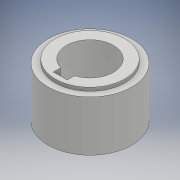
# Autodesk Inventor part: Outer Wheel Spacer
Saved by Autodesk Inventor 2018 (Build 220112000, 112)
## iProperties
Created: 2018-01-21
Part Number: Outer Wheel Spacer
Material: Generic
Document SubType Name: Modeling
Designer: Apple
Density: 1 g/cm^3
Appearance: Default
Author: Apple
Autodesk Inventor part; units mm, degrees
ref_plane "YZ Plane" through (0, 0, 0) normal (1, 0, 0) x (0, 1, 0)
ref_plane "XZ Plane" through (0, 0, 0) normal (0, 1, 0) x (-1, 0, 0)
ref_plane "XY Plane" through (0, 0, 0) normal (0, 0, 1) x (1, 0, 0)
sketch "Sketch1" plane through (0, 0, 0) normal (0, 0, 1) x (1, 0, 0)
  circle A0 centre (0, 0) radius 6.75
  circle A1 centre (0, 0) radius 12
  dimension "d0" = 13.5
  dimension "d1" = 24
  constraints: 2 centre point, 2 coincident
  measures "d0" diameter of A0
  measures "d1" diameter of A1
extrude "Extrusion1" add sketch "Sketch1" along normal blind 14.5
sketch "Sketch3" plane through (0, 0, 14.5) normal (0, 0, 1) x (1, 0, 0)
  circle A0 centre (0, 0) radius 10
  circle A1 centre (0, 0) radius 6.75 projected
  dimension "d7" = 20
  constraints: 1 centre point, 1 coincident
  measures "d7" diameter of A0
extrude "Extrusion3" add sketch "Sketch3" along normal blind 1
sketch "Sketch5" plane through (0, 0, 15.5) normal (0, 0, 1) x (1, 0, 0)
  line L0 (2, -8.55) -> (-2, -8.55)
  line L1 (-2, -8.55) -> (-2, -4.55)
  line L2 (-2, -4.55) -> (2, -4.55)
  line L3 (2, -4.55) -> (2, -8.55)
  line L4 (3.7816, -6.55) -> (-3.7816, -6.55) projected
  point P0 (0, 0)
  point P1 (0, -8.55)
  point P2 (-2, -6.55)
  point P3 (0, -6.55)
  dimension "d13" = 4
  dimension "d14" = 4
  constraints: 8 end point, 3 midpoint, 2 parallel, 1 horizontal, 1 horizontal alignment, 1 perpendicular, 1 vertical alignment
  measures "d13" distance of L0.start L0.end
  measures "d14" distance of L0.end L1.end
extrude "Extrusion5" cut sketch "Sketch5" against normal through all
body "Solid1"
